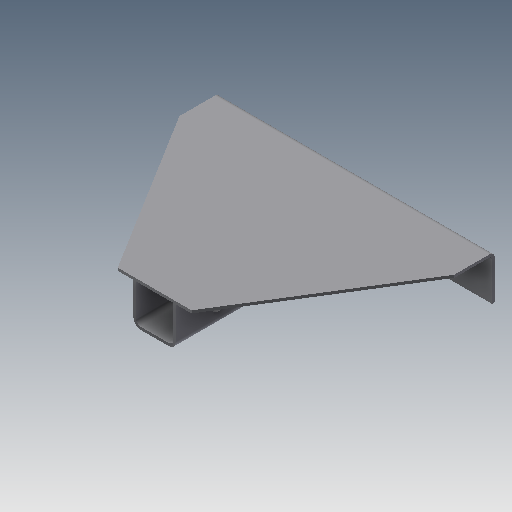
# Autodesk Inventor part: P2348-S1-Unistrut
Saved by Autodesk Inventor 2019.1 (Build 231200000, 200)
## iProperties
Created: 2009-08-10
Part Number: P2348-S1-Unistrut
Material: Generic
Document SubType Name: Sheet Metal
Designer: Demir Ali
Density: 1 g/cm^3
Sheet Metal Rule: Default_mm
Mass: 264.48 g
Surface Area: 1790.17 cm^2
Volume: 264.48 cm^3
Description: Unistrut Foot Plate
Stock Number: NA
Appearance: Default
Title: Purchased Part
Author: Demir Ali
Revision Number: A
Autodesk Inventor part; units mm, degrees
ref_plane "YZ Plane" through (0, 0, 0) normal (1, 0, 0) x (0, 1, 0)
ref_plane "XZ Plane" through (0, 0, 0) normal (0, 1, 0) x (-1, 0, 0)
ref_plane "XY Plane" through (0, 0, 0) normal (0, 0, 1) x (1, 0, 0)
sketch "Sketch1" plane through (0, 0, 0) normal (0, 0, 1) x (1, 0, 0)
  line L0 (-152.5, -24.5) -> (152.5, -24.5)
  line L1 (152.5, -24.5) -> (152.5, 24.5)
  line L2 (152.5, 24.5) -> (-152.5, 24.5)
  line L3 (-152.5, 24.5) -> (-152.5, -24.5)
  point P0 (0, 24.5)
  point P1 (0, 0)
  point P2 (-152.5, 0)
  point P3 (0, -24.5)
  dimension "d0" = 305
  dimension "d1" = 49
  measures "d0" distance of L1.end L2.end
  measures "d1" distance of L2.end L0.start
extrude "Plate1" add sketch "Sketch1" along normal blind 3
sketch "Sketch2" plane through (152.5, 21.5, 0) normal (0, 1, 0) x (-1, 0, 0)
  line L0 (305, 0) -> (0, 0)
  line L1 (0, 0) -> (0, -225)
  line L2 (0, -225) -> (305, -225)
  line L3 (305, -225) -> (305, 0)
  constraints: 6 end point, 1 horizontal, 1 perpendicular, 1 vertical
edge flange "Flange1" height 225 angle 90 thickness 3 bend radius 3 thickness toward (0, 1, 0) relief straight relief width 3 relief depth 1.5 edges at (0, 24.5, 0) wall of the first edge with corners at (-152.5, 21.5, 0) (152.5, 21.5, 0) (152.5, 21.5, 225) (-152.5, 21.5, 225)
bend "Bend1"
corner "Corner1"
chamfer "Corner Chamfer1" distance 111.5 distance2 180 1 edges at (-152.5, 23, 225) measured on face at (-152, 23, 225)
chamfer "Corner Chamfer2" distance 111.5 distance2 180 1 edges at (152.5, 23, 225) measured on face at (152, 23, 225)
sketch "Sketch4" plane through (0, 0, 3) normal (0, 0, 1) x (1, 0, 0)
  line L0 (152.5, -24.5) -> (-152.5, -24.5) projected
  line L1 (-112.5, 0) -> (112.5, 0)
  point P0 (0, 0)
  point P1 (0, 0)
  point P2 (0, -24.5)
  dimension "d26" = 225
  dimension "d27" = 24.5
  constraints: 2 end point, 2 midpoint, 1 parallel, 1 vertical alignment
  measures "d26" distance of L1.start L1.end
  measures "d27" distance between parallel lines of L0 L1
hole "Hole1" at (-112.5, 0, 3) direction (0, 0, -1) diameter 14 end through all
pattern_linear "Rectangular Pattern1" count 2 spacing 225 along (1, 0, 0) of "Hole1"
sketch "Sketch3" plane through (-41, 21.5, 225) normal (0, 0, 1) x (1, 0, 0)
  line L0 (0, 0) -> (82, 0) projected
  line L1 (20.5, -41) -> (61.5, -41)
  line L2 (61.5, -41) -> (61.5, 0)
  line L3 (61.5, 0) -> (20.5, 0)
  line L4 (20.5, 0) -> (20.5, -41)
  line L5 (17.5, 0) -> (17.5, -44)
  line L6 (17.5, -44) -> (64.5, -44)
  line L7 (64.5, -44) -> (64.5, 0)
  point P0 (41, -21.5)
  point P1 (41, 0)
  dimension "d19" = 41
  dimension "d20" = 41
  dimension "d21" = 3
  dimension "d22" = 3
  dimension "d23" = 3
  constraints: 14 end point, 3 parallel, 3 perpendicular, 2 midpoint, 2 point on line, 1 horizontal
  measures "d19" distance of L3.end L1.start
  measures "d20" distance of L1.start L1.end
  measures "d21" distance between parallel lines of L1 L6
  measures "d22" distance between parallel lines of L4 L5
  measures "d23" distance between parallel lines of L7 L2
extrude "Extrusion1" add sketch "Sketch3" against normal up to next contours L0 L4 L1 L2 L7 L6 L5
fillet "Fillet1" radius 5 2 edges at (-20.5, -19.5, 114) (20.5, -19.5, 114)
fillet "Fillet1" radius 8 2 edges at (-23.5, -22.5, 114) (23.5, -22.5, 114)
hole "Hole2" at (23.5, -2, 28) direction (-1, 0, 0) diameter 14 depth 20 tip angle 118
pattern_linear "Rectangular Pattern2" count 2 spacing 150 along (0, 0, 1) of "Hole2"
pattern_circular "Circular Pattern1" count 3 over 180 about axis through (0, 0, -10) along (0, 0, -1) of "Hole2", "Rectangular Pattern2"
equation "\"d33\" = Thickness"
equation "\"d37\" = d26"
equation "\"d20\" = d19"
equation "\"d21\" = Thickness"
equation "\"d22\" = Thickness"
equation "\"d23\" = Thickness"
equation "\"d55\" = Thickness"
equation "\"d3\" = BendReliefWidth"
equation "\"d4\" = BendReliefDepth"
equation "\"d5\" = MinimumRemnant"
equation "\"d6\" = BendRadius"
equation "\"d9\" = BendRadius"
equation "\"d10\" = CornerReliefSize"
equation "\"d11\" = GapSize"
equation "\"d12\" = JacobiRadiusSize"
equation "\"BendRadius\" = Thickness"
equation "\"BendReliefWidth\" = Thickness"
equation "\"BendReliefDepth\" = 0.5 * Thickness"
equation "\"CornerReliefSize\" = 4 * Thickness"
equation "\"MinimumRemnant\" = 2 * Thickness"
equation "\"TransitionRadius\" = BendRadius"
equation "\"JacobiRadiusSize\" = BendRadius"
equation "\"GapSize\" = Thickness"
equation "\"d2\" = BendRadius"
equation "\"Thickness\" = 3"
body "Solid1"
